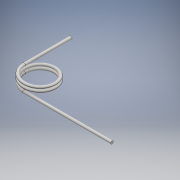
# Autodesk Inventor part: Coil
Saved by Autodesk Inventor 2016 (Build 200138000, 138)
## iProperties
Created: 2016-11-05
Part Number: Coil
Material: Generic
Document SubType Name: Modeling
Designer: Muhammad
Density: 1 g/cm^3
Appearance: Chrome - Polished
Author: Muhammad
Autodesk Inventor part; units mm, degrees
ref_plane "YZ Plane" through (0, 0, 0) normal (1, 0, 0) x (0, 1, 0)
ref_plane "XZ Plane" through (0, 0, 0) normal (0, 1, 0) x (-1, 0, 0)
ref_plane "XY Plane" through (0, 0, 0) normal (0, 0, 1) x (1, 0, 0)
sketch "Sketch1" plane through (0, 0, 0) normal (0, 1, 0) x (-1, 0, 0)
  line L0 (0, 0) -> (5.5, 0)
  circle A0 centre (5.5, 0) radius 0.5
  line L1 (0, 0) -> (0, -0.669)
  dimension "d2" = 5.5
  dimension "d3" = 1
  constraints: 4 end point, 1 centre point, 1 coincident, 1 horizontal, 1 vertical
  measures "d2" distance of L0.start L0.end
  measures "d3" diameter of A0
coil "Coil1" sketch "Sketch1" operation add axis through (0, 0, 0) along (0, 0, 1) pitch 1.25 turns 2 hand left
sketch "Sketch2" plane through (-5.5, 0, 2.5) normal (0, 1, 0) x (1, 0, 0)
  circle A0 centre (0, 0) radius 0.5
  point P0 (5.5, 2.5)
  constraints: 1 centre point
extrude "Extrusion1" add sketch "Sketch2" along normal blind 17
sketch "Sketch3" plane through (-5.5, 0, 0) normal (0, -1, 0) x (1, 0, 0)
  circle A0 centre (0, 0) radius 0.5
  line L0 (0, 0) -> (5.5, 0)
  line L1 (5.5, 0) -> (5.5, 1.9866)
  constraints: 4 end point, 1 centre point, 1 horizontal, 1 perpendicular
coil "Coil2" sketch "Sketch3" operation add axis through (0, 0, 0) along (0, 0, -1) pitch 2 turns 0.25 hand left
sketch "Sketch4" plane through (0, -5.5, -0.5) normal (1, 0, 0) x (0, 0, -1)
  circle A0 centre (0, 0) radius 0.5 projected
  circle A1 centre (0, 0) radius 0.5
  point P0 (-0.5, 5.5)
  point P1 (0, 0.5)
  constraints: 1 centre point, 1 coincident, 1 vertical alignment
extrude "Extrusion2" add sketch "Sketch4" along normal blind 32
body "Solid1"
